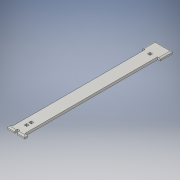
# Autodesk Inventor part: Arm Top
Saved by Autodesk Inventor 2016 (Build 200138000, 138)
## iProperties
Created: 2016-04-25
Part Number: Arm Top
Material: PVC-Piping
Document SubType Name: Modeling
Designer: rubenjm
Density: 1.4 g/cm^3
Appearance: Smooth - White
Author: rubenjm
Autodesk Inventor part; units mm, degrees
ref_plane "YZ Plane" through (0, 0, 0) normal (1, 0, 0) x (0, 1, 0)
ref_plane "XZ Plane" through (0, 0, 0) normal (0, 1, 0) x (-1, 0, 0)
ref_plane "XY Plane" through (0, 0, 0) normal (0, 0, 1) x (1, 0, 0)
sketch "Sketch1" plane through (0, 0, 0) normal (0, 1, 0) x (-1, 0, 0)
  line L0 (0, 0) -> (88.9, 0)
  line L1 (88.9, 0) -> (76.2, 0) construction
  line L2 (76.2, 0) -> (76.2, -12.7) construction
  line L3 (76.2, -12.7) -> (88.9, -12.7) construction
  line L4 (88.9, -12.7) -> (88.9, 0) construction
  line L5 (0, -349.25) -> (88.9, -349.25) construction
  line L6 (88.9, -698.5) -> (76.2, -698.5) construction
  line L7 (76.2, -698.5) -> (76.2, -685.8) construction
  line L8 (76.2, -685.8) -> (88.9, -685.8) construction
  line L9 (0, 0) -> (12.7, 0) construction
  line L10 (12.7, 0) -> (12.7, -12.7) construction
  line L11 (12.7, -12.7) -> (0, -12.7) construction
  line L12 (0, -12.7) -> (0, 0) construction
  line L13 (0, -698.5) -> (12.7, -698.5) construction
  line L14 (12.7, -698.5) -> (12.7, -685.8) construction
  line L15 (12.7, -685.8) -> (0, -685.8) construction
  line L16 (88.9, -12.7) -> (76.2, -12.7)
  line L17 (76.2, -12.7) -> (76.2, -685.8)
  line L18 (76.2, -685.8) -> (88.9, -685.8)
  line L19 (12.7, -685.8) -> (0, -685.8)
  line L20 (0, -12.7) -> (12.7, -12.7)
  line L21 (12.7, -12.7) -> (12.7, -685.8)
  line L22 (0, -12.7) -> (0, 0)
  line L23 (88.9, 0) -> (88.9, -12.7)
  line L24 (0, -685.8) -> (0, -749.3)
  line L25 (0, -749.3) -> (88.9, -749.3)
  line L26 (88.9, -749.3) -> (88.9, -685.8)
  dimension "d2" = 12.7
  dimension "d3" = 12.7
  dimension "d8" = 88.9
  dimension "d10" = 63.5
  constraints: 54 end point, 6 parallel, 4 horizontal, 3 perpendicular, 3 symmetric about line, 1 point on line
  measures "d2" distance of L3.end L2.end
  measures "d3" distance of L2.end L1.end
  measures "d8" distance of L25.end L24.end
  measures "d10" distance of L15.end L24.end
extrude "Extrusion1" add sketch "Sketch1" along normal blind 12.7
fillet "Fillet1" radius 6.35 3 edges at (-44.45, 12.7, 0) (-88.9, 12.7, -6.35) (0, 12.7, -6.35)
fillet "Fillet3" radius 6.35 3 edges at (-44.45, 12.7, -749.3) (-88.9, 12.7, -717.55) (0, 12.7, -717.55)
sketch "Sketch2" plane through (0, 12.7, 0) normal (0, 1, 0) x (1, 0, 0)
  line L0 (-88.9, 749.3) -> (0, 749.3) construction
  line L1 (-44.45, 749.3) -> (-44.45, 685.8) construction
  line L2 (-44.45, 749.3) -> (19.05, 749.3) construction
  line L3 (-44.45, 685.8) -> (-50.8, 685.8) construction
  line L4 (-44.45, 685.8) -> (-38.1, 685.8) construction
  line L5 (-50.8, 685.8) -> (-38.1, 685.8)
  line L6 (-38.1, 685.8) -> (-38.1, 673.1)
  line L7 (-38.1, 673.1) -> (-50.8, 673.1)
  line L8 (-50.8, 673.1) -> (-50.8, 685.8)
  line L9 (-44.45, 673.1) -> (-44.45, 82.55) construction
  line L10 (-44.45, 673.1) -> (546.1, 673.1) construction
  line L11 (-44.45, 82.55) -> (-50.8, 82.55) construction
  line L12 (-44.45, 82.55) -> (-38.1, 82.55) construction
  line L13 (-50.8, 82.55) -> (-38.1, 82.55)
  line L14 (-38.1, 82.55) -> (-38.1, 69.85)
  line L15 (-38.1, 69.85) -> (-50.8, 69.85)
  line L16 (-50.8, 69.85) -> (-50.8, 82.55)
  line L17 (-44.45, 69.85) -> (-44.45, 59.944) construction
  line L18 (-44.45, 69.85) -> (-34.544, 69.85) construction
  line L19 (-44.45, 59.944) -> (-50.8, 59.944) construction
  line L20 (-44.45, 59.944) -> (-38.1, 59.944) construction
  line L21 (-50.8, 59.944) -> (-38.1, 59.944)
  line L22 (-38.1, 59.944) -> (-38.1, 47.244)
  line L23 (-38.1, 47.244) -> (-50.8, 47.244)
  line L24 (-50.8, 47.244) -> (-50.8, 59.944)
  line L25 (-44.45, 47.244) -> (-44.45, 0) construction
  line L26 (-88.9, 0) -> (0, 0) construction
  line L27 (-44.45, 0) -> (-38.1, 0) construction
  line L28 (-44.45, 0) -> (-38.1, 0) construction
  line L29 (-38.1, 0) -> (-50.8, 0)
  line L30 (-50.8, 0) -> (-50.8, 12.7)
  line L31 (-50.8, 12.7) -> (-38.1, 12.7)
  line L32 (-38.1, 12.7) -> (-38.1, 0)
  dimension "d12" = 63.5
  dimension "d13" = 90
  dimension "d14" = 6.35
  dimension "d15" = 180
  dimension "d16" = 12.7
  dimension "d17" = 12.7
  dimension "d18" = 590.55
  dimension "d19" = 90
  dimension "d20" = 6.35
  dimension "d21" = 180
  dimension "d22" = 12.7
  dimension "d23" = 12.7
  dimension "d24" = 9.906
  dimension "d25" = 90
  dimension "d26" = 6.35
  dimension "d27" = 180
  dimension "d28" = 12.7
  dimension "d29" = 12.7
  dimension "d30" = 6.35
  dimension "d31" = 0
  dimension "d32" = 12.7
  dimension "d33" = 12.7
  constraints: 62 end point, 15 horizontal, 8 parallel, 7 equal length, 5 midpoint, 4 perpendicular, 3 vertical
  measures "d12" distance of L1.start L1.end
  measures "d13" angle of L1 L2
  measures "d14" distance of L1.end L3.end
  measures "d15" angle of L3 L4
  measures "d16" distance of L6.end L7.end
  measures "d17" distance of L5.end L6.end
  measures "d18" distance of L9.start L9.end
  measures "d19" angle of L9 L10
  measures "d20" distance of L9.end L11.end
  measures "d21" angle of L11 L12
  measures "d22" distance of L14.end L15.end
  measures "d23" distance of L13.end L14.end
  measures "d24" distance of L17.start L17.end
  measures "d25" angle of L17 L18
  measures "d26" distance of L17.end L19.end
  measures "d27" angle of L19 L20
  measures "d28" distance of L22.end L23.end
  measures "d29" distance of L21.end L22.end
  measures "d30" distance of L25.end L27.end
  measures "d31" distance between parallel lines of L27 L28
  measures "d32" distance of L30.end L31.end
  measures "d33" distance of L29.end L30.end
extrude "Extrusion2" cut sketch "Sketch2" along normal through all both and the other way through all
body "Solid1"
